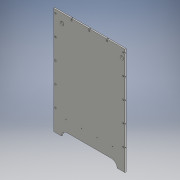
# Autodesk Inventor part: Venstre
Saved by Autodesk Inventor 2016 (Build 200138000, 138)
## iProperties
Created: 2016-02-23
Part Number: Venstre
Material: Generic
Document SubType Name: Modeling
Designer: Mathias L. Kjeldgaard
Density: 1 g/cm^3
Appearance: Default
Author: Mathias L. Kjeldgaard
Autodesk Inventor part; units mm, degrees
ref_plane "YZ Plane" through (0, 0, 0) normal (1, 0, 0) x (0, 1, 0)
ref_plane "XZ Plane" through (0, 0, 0) normal (0, 1, 0) x (-1, 0, 0)
ref_plane "XY Plane" through (0, 0, 0) normal (0, 0, 1) x (1, 0, 0)
sketch "Sketch1" plane through (0, 0, 0) normal (0, 1, 0) x (-1, 0, 0)
  line L0 (160, 240) -> (-160, 240)
  line L1 (-160, 240) -> (-160, -240)
  line L2 (-160, -240) -> (160, -240)
  line L3 (160, -240) -> (160, 240)
  point P0 (0, 0)
  dimension "d0" = 320
  dimension "d1" = 480
  dimension "d2" = 160
  dimension "d3" = 240
  constraints: 8 end point, 2 parallel, 1 horizontal, 1 perpendicular
  measures "d0" distance of L2.end L1.end
  measures "d1" distance of L1.end L0.end
  measures "d2" distance from line of L1 point (0, 0)
  measures "d3" distance from line of L2 point (0, 0)
extrude "Tykkelsen" add sketch "Sketch1" along normal mid plane 6
sketch "Sketch2" plane through (0, -3, 0) normal (0, -1, 0) x (1, 0, 0)
  line L0 (160, -240) -> (-160, -240) projected
  arc A0 (-100, -215) -> (-125, -240) centre (-100, -240) ccw
  arc A1 (125, -240) -> (100, -215) centre (100, -240) ccw
  line L1 (100, -215) -> (-100, -215)
  line L2 (100, -240) -> (-100, -240)
  point P0 (0, 0)
  dimension "d6" = 50
  dimension "d7" = 50
  dimension "d8" = 60
  dimension "d9" = 60
  constraints: 4 end point, 4 point on circle, 4 point on line, 2 centre point, 2 tangent, 1 collinear
  measures "d6" diameter of A0
  measures "d7" diameter of A1
  measures "d8" distance of L0.end L2.end
  measures "d9" distance of L0.start L2.start
extrude "Fødder" cut sketch "Sketch2" against normal up to next
sketch "Sketch3" plane through (-0.7023, -3, -0.8181) normal (0, 1, 0) x (1, 0, 0)
  line L0 (152.9023, 140.4319) -> (151.5023, 140.4319)
  line L1 (160.7023, 141.6819) -> (154.3813, 141.6819)
  arc A0 (152.9023, 140.4319) -> (154.3813, 141.6819) centre (152.9023, 141.9319) ccw
  arc A1 (150.0043, 141.8542) -> (151.5023, 140.4319) centre (151.5023, 141.9319) ccw
  line L2 (160.7023, 144.6819) -> (154.3813, 144.6819)
  arc A2 (150.0043, 144.5096) -> (150.0043, 141.8542) centre (150.7023, 143.1819) ccw
  arc A3 (154.3813, 144.6819) -> (152.9023, 145.9319) centre (152.9023, 144.4319) ccw
  arc A4 (151.5023, 145.9319) -> (150.0043, 144.5096) centre (151.5023, 144.4319) ccw
  line L3 (151.5023, 145.9319) -> (152.9023, 145.9319)
  line L4 (160.7023, 141.6819) -> (160.7023, 144.6819)
  line L5 (150.7023, 143.1819) -> (160.7023, 143.1819) construction
  line L6 (77.9523, -233.0181) -> (77.9523, -231.6181)
  line L7 (79.2023, -240.8181) -> (79.2023, -234.4971)
  arc A5 (77.9523, -233.0181) -> (79.2023, -234.4971) centre (79.4523, -233.0181) ccw
  arc A6 (79.3746, -230.1201) -> (77.9523, -231.6181) centre (79.4523, -231.6181) ccw
  arc A7 (82.03, -230.1201) -> (79.3746, -230.1201) centre (80.7023, -230.8181) ccw
  arc A8 (83.4523, -231.6181) -> (82.03, -230.1201) centre (81.9523, -231.6181) ccw
  line L8 (83.4523, -231.6181) -> (83.4523, -233.0181)
  line L9 (82.2023, -240.8181) -> (82.2023, -234.4971)
  line L10 (80.7023, -232.1889) -> (80.7023, -240) construction
  line L11 (79.2023, -240.8181) -> (82.2023, -240.8181)
  arc A9 (82.2023, -234.4971) -> (83.4523, -233.0181) centre (81.9523, -233.0181) ccw
  line L12 (-2.0477, -233.0181) -> (-2.0477, -231.6181)
  line L13 (-0.7977, -240.8181) -> (-0.7977, -234.4971)
  arc A10 (-2.0477, -233.0181) -> (-0.7977, -234.4971) centre (-0.5477, -233.0181) ccw
  arc A11 (-0.6254, -230.1201) -> (-2.0477, -231.6181) centre (-0.5477, -231.6181) ccw
  arc A12 (2.03, -230.1201) -> (-0.6254, -230.1201) centre (0.7023, -230.8181) ccw
  arc A13 (3.4523, -231.6181) -> (2.03, -230.1201) centre (1.9523, -231.6181) ccw
  line L14 (3.4523, -231.6181) -> (3.4523, -233.0181)
  line L15 (2.2023, -240.8181) -> (2.2023, -234.4971)
  line L16 (0.7023, -230.8181) -> (0.7023, -240) construction
  line L17 (-0.7977, -240.8181) -> (2.2023, -240.8181)
  arc A14 (2.2023, -234.4971) -> (3.4523, -233.0181) centre (1.9523, -233.0181) ccw
  arc A15 (152.9023, 48.4319) -> (154.3813, 49.6819) centre (152.9023, 49.9319) ccw
  line L18 (150.7023, 51.1819) -> (160.7023, 51.1819) construction
  arc A16 (151.5023, 53.9319) -> (150.0043, 52.5096) centre (151.5023, 52.4319) ccw
  arc A17 (150.0043, 49.8542) -> (151.5023, 48.4319) centre (151.5023, 49.9319) ccw
  arc A18 (150.0043, 52.5096) -> (150.0043, 49.8542) centre (150.7023, 51.1819) ccw
  line L19 (160.7023, 49.6819) -> (154.3813, 49.6819)
  line L20 (151.5023, 53.9319) -> (152.9023, 53.9319)
  arc A19 (154.3813, 52.6819) -> (152.9023, 53.9319) centre (152.9023, 52.4319) ccw
  line L21 (160.7023, 52.6819) -> (154.3813, 52.6819)
  line L22 (152.9023, 48.4319) -> (151.5023, 48.4319)
  line L23 (160.7023, 49.6819) -> (160.7023, 52.6819)
  arc A20 (152.9023, -43.5681) -> (154.3813, -42.3181) centre (152.9023, -42.0681) ccw
  line L24 (150.7023, -40.8181) -> (160.7023, -40.8181) construction
  arc A21 (151.5023, -38.0681) -> (150.0043, -39.4904) centre (151.5023, -39.5681) ccw
  arc A22 (150.0043, -42.1458) -> (151.5023, -43.5681) centre (151.5023, -42.0681) ccw
  arc A23 (150.0043, -39.4904) -> (150.0043, -42.1458) centre (150.7023, -40.8181) ccw
  line L25 (160.7023, -42.3181) -> (154.3813, -42.3181)
  line L26 (151.5023, -38.0681) -> (152.9023, -38.0681)
  arc A24 (154.3813, -39.3181) -> (152.9023, -38.0681) centre (152.9023, -39.5681) ccw
  line L27 (160.7023, -39.3181) -> (154.3813, -39.3181)
  line L28 (152.9023, -43.5681) -> (151.5023, -43.5681)
  line L29 (160.7023, -42.3181) -> (160.7023, -39.3181)
  arc A25 (152.9023, -135.5681) -> (154.3813, -134.3181) centre (152.9023, -134.0681) ccw
  line L30 (150.7023, -132.8181) -> (160.7023, -132.8181) construction
  arc A26 (151.5023, -130.0681) -> (150.0043, -131.4904) centre (151.5023, -131.5681) ccw
  arc A27 (150.0043, -134.1458) -> (151.5023, -135.5681) centre (151.5023, -134.0681) ccw
  arc A28 (150.0043, -131.4904) -> (150.0043, -134.1458) centre (150.7023, -132.8181) ccw
  line L31 (160.7023, -134.3181) -> (154.3813, -134.3181)
  line L32 (151.5023, -130.0681) -> (152.9023, -130.0681)
  arc A29 (154.3813, -131.3181) -> (152.9023, -130.0681) centre (152.9023, -131.5681) ccw
  line L33 (160.7023, -131.3181) -> (154.3813, -131.3181)
  line L34 (152.9023, -135.5681) -> (151.5023, -135.5681)
  line L35 (160.7023, -134.3181) -> (160.7023, -131.3181)
  arc A30 (152.9023, -227.5681) -> (154.3813, -226.3181) centre (152.9023, -226.0681) ccw
  line L36 (150.7023, -224.8181) -> (160.7023, -224.8181) construction
  arc A31 (151.5023, -222.0681) -> (150.0043, -223.4904) centre (151.5023, -223.5681) ccw
  arc A32 (150.0043, -226.1458) -> (151.5023, -227.5681) centre (151.5023, -226.0681) ccw
  arc A33 (150.0043, -223.4904) -> (150.0043, -226.1458) centre (150.7023, -224.8181) ccw
  line L37 (160.7023, -226.3181) -> (154.3813, -226.3181)
  line L38 (151.5023, -222.0681) -> (152.9023, -222.0681)
  arc A34 (154.3813, -223.3181) -> (152.9023, -222.0681) centre (152.9023, -223.5681) ccw
  line L39 (160.7023, -223.3181) -> (154.3813, -223.3181)
  line L40 (152.9023, -227.5681) -> (151.5023, -227.5681)
  line L41 (160.7023, -226.3181) -> (160.7023, -223.3181)
  line L42 (0.7023, 0.5064) -> (0.7023, -145.6554) construction
  line L43 (-99.2977, 214.1819) -> (100.7023, 214.1819) projected
  line L44 (160.7023, 239.1819) -> (160.7023, -240.8181) projected
  line L45 (125.7023, 239.1819) -> (160.7023, 239.1819) projected
  line L46 (160.7023, -240.8181) -> (-159.2977, -240.8181) projected
  line L47 (-151.4977, 140.4319) -> (-150.0977, 140.4319)
  line L48 (-159.2977, 141.6819) -> (-152.9768, 141.6819)
  arc A35 (-152.9768, 141.6819) -> (-151.4977, 140.4319) centre (-151.4977, 141.9319) ccw
  arc A36 (-150.0977, 140.4319) -> (-148.5998, 141.8542) centre (-150.0977, 141.9319) ccw
  line L49 (-159.2977, 144.6819) -> (-152.9768, 144.6819)
  arc A37 (-148.5998, 141.8542) -> (-148.5998, 144.5096) centre (-149.2977, 143.1819) ccw
  arc A38 (-151.4977, 145.9319) -> (-152.9768, 144.6819) centre (-151.4977, 144.4319) ccw
  arc A39 (-148.5998, 144.5096) -> (-150.0977, 145.9319) centre (-150.0977, 144.4319) ccw
  line L50 (-150.0977, 145.9319) -> (-151.4977, 145.9319)
  line L51 (-159.2977, 141.6819) -> (-159.2977, 144.6819)
  line L52 (-149.2977, 143.1819) -> (-159.2977, 143.1819) construction
  line L53 (-76.5477, -233.0181) -> (-76.5477, -231.6181)
  line L54 (-77.7977, -240.8181) -> (-77.7977, -234.4971)
  arc A40 (-77.7977, -234.4971) -> (-76.5477, -233.0181) centre (-78.0477, -233.0181) ccw
  arc A41 (-76.5477, -231.6181) -> (-77.97, -230.1201) centre (-78.0477, -231.6181) ccw
  arc A42 (-77.97, -230.1201) -> (-80.6254, -230.1201) centre (-79.2977, -230.8181) ccw
  arc A43 (-80.6254, -230.1201) -> (-82.0477, -231.6181) centre (-80.5477, -231.6181) ccw
  line L55 (-82.0477, -231.6181) -> (-82.0477, -233.0181)
  line L56 (-80.7977, -240.8181) -> (-80.7977, -234.4971)
  line L57 (-79.2977, -232.1889) -> (-79.2977, -240) construction
  line L58 (-77.7977, -240.8181) -> (-80.7977, -240.8181)
  arc A44 (-82.0477, -233.0181) -> (-80.7977, -234.4971) centre (-80.5477, -233.0181) ccw
  arc A45 (-152.9768, 49.6819) -> (-151.4977, 48.4319) centre (-151.4977, 49.9319) ccw
  line L59 (-149.2977, 51.1819) -> (-159.2977, 51.1819) construction
  arc A46 (-148.5998, 52.5096) -> (-150.0977, 53.9319) centre (-150.0977, 52.4319) ccw
  arc A47 (-150.0977, 48.4319) -> (-148.5998, 49.8542) centre (-150.0977, 49.9319) ccw
  arc A48 (-148.5998, 49.8542) -> (-148.5998, 52.5096) centre (-149.2977, 51.1819) ccw
  line L60 (-159.2977, 49.6819) -> (-152.9768, 49.6819)
  line L61 (-150.0977, 53.9319) -> (-151.4977, 53.9319)
  arc A49 (-151.4977, 53.9319) -> (-152.9768, 52.6819) centre (-151.4977, 52.4319) ccw
  line L62 (-159.2977, 52.6819) -> (-152.9768, 52.6819)
  line L63 (-151.4977, 48.4319) -> (-150.0977, 48.4319)
  line L64 (-159.2977, 49.6819) -> (-159.2977, 52.6819)
  arc A50 (-152.9768, -42.3181) -> (-151.4977, -43.5681) centre (-151.4977, -42.0681) ccw
  line L65 (-149.2977, -40.8181) -> (-159.2977, -40.8181) construction
  arc A51 (-148.5998, -39.4904) -> (-150.0977, -38.0681) centre (-150.0977, -39.5681) ccw
  arc A52 (-150.0977, -43.5681) -> (-148.5998, -42.1458) centre (-150.0977, -42.0681) ccw
  arc A53 (-148.5998, -42.1458) -> (-148.5998, -39.4904) centre (-149.2977, -40.8181) ccw
  line L66 (-159.2977, -42.3181) -> (-152.9768, -42.3181)
  line L67 (-150.0977, -38.0681) -> (-151.4977, -38.0681)
  arc A54 (-151.4977, -38.0681) -> (-152.9768, -39.3181) centre (-151.4977, -39.5681) ccw
  line L68 (-159.2977, -39.3181) -> (-152.9768, -39.3181)
  line L69 (-151.4977, -43.5681) -> (-150.0977, -43.5681)
  line L70 (-159.2977, -42.3181) -> (-159.2977, -39.3181)
  arc A55 (-152.9768, -134.3181) -> (-151.4977, -135.5681) centre (-151.4977, -134.0681) ccw
  line L71 (-149.2977, -132.8181) -> (-159.2977, -132.8181) construction
  arc A56 (-148.5998, -131.4904) -> (-150.0977, -130.0681) centre (-150.0977, -131.5681) ccw
  arc A57 (-150.0977, -135.5681) -> (-148.5998, -134.1458) centre (-150.0977, -134.0681) ccw
  arc A58 (-148.5998, -134.1458) -> (-148.5998, -131.4904) centre (-149.2977, -132.8181) ccw
  line L72 (-159.2977, -134.3181) -> (-152.9768, -134.3181)
  line L73 (-150.0977, -130.0681) -> (-151.4977, -130.0681)
  arc A59 (-151.4977, -130.0681) -> (-152.9768, -131.3181) centre (-151.4977, -131.5681) ccw
  line L74 (-159.2977, -131.3181) -> (-152.9768, -131.3181)
  line L75 (-151.4977, -135.5681) -> (-150.0977, -135.5681)
  line L76 (-159.2977, -134.3181) -> (-159.2977, -131.3181)
  arc A60 (-152.9768, -226.3181) -> (-151.4977, -227.5681) centre (-151.4977, -226.0681) ccw
  line L77 (-149.2977, -224.8181) -> (-159.2977, -224.8181) construction
  arc A61 (-148.5998, -223.4904) -> (-150.0977, -222.0681) centre (-150.0977, -223.5681) ccw
  arc A62 (-150.0977, -227.5681) -> (-148.5998, -226.1458) centre (-150.0977, -226.0681) ccw
  arc A63 (-148.5998, -226.1458) -> (-148.5998, -223.4904) centre (-149.2977, -224.8181) ccw
  line L78 (-159.2977, -226.3181) -> (-152.9768, -226.3181)
  line L79 (-150.0977, -222.0681) -> (-151.4977, -222.0681)
  arc A64 (-151.4977, -222.0681) -> (-152.9768, -223.3181) centre (-151.4977, -223.5681) ccw
  line L80 (-159.2977, -223.3181) -> (-152.9768, -223.3181)
  line L81 (-151.4977, -227.5681) -> (-150.0977, -227.5681)
  line L82 (-159.2977, -226.3181) -> (-159.2977, -223.3181)
  line L83 (-159.2977, 239.1819) -> (-159.2977, -240.8181)
  line L84 (-159.2977, -240.8181) -> (160.7023, -240.8181)
  point P0 (0.8017, -240.8181)
  point P1 (80.7023, -240.8181)
  point P2 (0.7023, 215)
  point P3 (0.7023, 214.1819)
  point P4 (-79.2977, -240.8181)
  dimension "d27" = 1.5
  dimension "d26" = 1.25
  dimension "d28" = 4.25
  dimension "d25" = 6.321
  dimension "d24" = 9.2
  dimension "d23" = 9.2
  dimension "d22" = 10
  dimension "d13" = 92
  dimension "d19" = 80
  dimension "d52" = 96
  dimension "d53" = 1.5
  dimension "d54" = 80
  dimension "d55" = 7.8
  dimension "d56" = 1.4
  dimension "d57" = 0.8
  dimension "d59" = 7.8
  dimension "d60" = 0.8
  dimension "d61" = 1.4
  constraints: 162 end point, 132 point on circle, 102 symmetric about line, 65 centre point, 18 tangent, 14 equal radius, 13 parallel, 8 point on line, 5 midpoint, 3 perpendicular, 3 vertical alignment, 2 horizontal alignment, 1 collinear, 1 horizontal, 1 vertical, 137 other
  measures "d27" radius of A3
  measures "d26" distance between parallel lines of L2 L3
  measures "d28" distance between parallel lines of L0 L2
  measures "d25" distance from line of L2.end L4
  measures "d24" distance from line of L3.start L4
  measures "d23" distance from line of A1.centre L4
  measures "d22" distance from line of L5.start L4
  measures "d13" distance of A0.centre A15.centre
  measures "d19" distance between parallel lines of L16 L10
  measures "d52" distance between parallel lines of L45 L5
  measures "d53" radius of A4
  measures "d54" distance between parallel lines of L44 L10
  measures "d55" distance from line of A9.centre L11
  measures "d56" distance of A8.centre A9.centre
  measures "d57" vertical distance of A8.centre A7.centre
  measures "d59" distance from line of A14.centre L17
  measures "d60" vertical distance of A13.centre L16.start
  measures "d61" distance of A14.centre A13.centre
extrude "Monteringshuller" cut sketch "Sketch3" along normal blind 5
sketch "Sketch8" plane through (0, -3, 0) normal (0, -1, 0) x (1, 0, 0)
  circle A0 centre (-122, 200) radius 8
  circle A1 centre (147, 200) radius 8
  line L0 (-160, -240) -> (-160, 240) projected
  line L1 (-160, 240) -> (160, 240) projected
  line L2 (160, 240) -> (160, -240) projected
  point P0 (0, 0)
  dimension "d75" = 16
  dimension "d76" = 16
  dimension "d77" = 38
  dimension "d78" = 40
  dimension "d79" = 13
  dimension "d80" = 40
  constraints: 2 centre point
  measures "d75" diameter of A0
  measures "d76" diameter of A1
  measures "d77" distance from line of L0 A0.centre
  measures "d78" distance from line of L1 A0.centre
  measures "d79" distance from line of L2 A1.centre
  measures "d80" distance from line of L1 A1.centre
extrude "Leje Huller" cut sketch "Sketch8" against normal blind 3.5
sketch "Sketch9" plane through (0, -3, 0) normal (0, -1, 0) x (1, 0, 0)
  line L0 (0, 0) -> (0, -101.4818) construction
  line L1 (218.4597, -166) -> (-162.3723, -166) construction
  line L2 (125, -240) -> (160, -240) projected
  circle A0 centre (105, -166) radius 1.5
  circle A1 centre (35, -166) radius 1.5
  circle A2 centre (-35, -166) radius 1.5
  circle A3 centre (-105, -166) radius 1.5
  dimension "d90" = 74
  dimension "d94" = 55
  dimension "d95" = 3
  dimension "d98" = 70
  constraints: 4 centre point, 4 end point, 1 horizontal, 1 point on line, 1 vertical, 6 other
  measures "d90" distance between parallel lines of L2 L1
  measures "d94" horizontal distance of L2.end A0.centre
  measures "d95" diameter of A0
  measures "d98" distance of A0.centre A1.centre
extrude "Mellemplade monteringshuller" cut sketch "Sketch9" against normal blind 10
equation "\"d2\" = 0.5 * d0"
equation "\"d3\" = 0.5 * d1"
equation "\"d76\" = d75"
body "Solid1"
